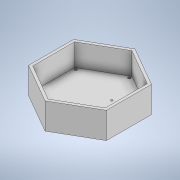
# Autodesk Inventor part: Improved Internal Base
Saved by Autodesk Inventor 2020 (Build 240168000, 168)
## iProperties
Created: 2020-02-13
Part Number: Improved Internal Base
Material: Generic
Document SubType Name: Modeling
Designer: danie
Density: 1 g/cm^3
Appearance: Default
Author: danie
Autodesk Inventor part; units mm, degrees
ref_plane "YZ Plane" through (0, 0, 0) normal (1, 0, 0) x (0, 1, 0)
ref_plane "XZ Plane" through (0, 0, 0) normal (0, 1, 0) x (-1, 0, 0)
ref_plane "XY Plane" through (0, 0, 0) normal (0, 0, 1) x (1, 0, 0)
sketch "Sketch1" plane through (0, 0, 0) normal (0, 1, 0) x (-1, 0, 0)
  line L0 (0, 0) -> (0, -80)
  line L1 (0, -80) -> (69.282, -120)
  line L2 (69.282, -120) -> (138.5641, -80)
  line L3 (138.5641, -80) -> (138.5641, 0)
  line L4 (138.5641, 0) -> (69.282, 40)
  line L5 (69.282, 40) -> (0, 0)
  line L6 (-5, 2.8868) -> (-5, -82.8868)
  line L7 (-5, -82.8868) -> (69.282, -125.7735)
  line L8 (69.282, -125.7735) -> (143.5641, -82.8868)
  line L9 (143.5641, -82.8868) -> (143.5641, 2.8868)
  line L10 (143.5641, 2.8868) -> (69.282, 45.7735)
  line L11 (69.282, 45.7735) -> (-5, 2.8868)
  line L12 (0, 0) -> (-5, 0) construction
  line L13 (-5, 2.8868) -> (0, 0) construction
  dimension "wall" = 80
  dimension "d1" = 80
  dimension "d2" = 80
  dimension "d3" = 80
  dimension "d4" = 80
  dimension "d5" = 80
  dimension "d6" = 120
  dimension "d7" = 120
  dimension "d9" = 120
  dimension "d10" = 120
  dimension "d11" = 120
  dimension "wallThickness" = 5
  dimension "d15" = 5
  dimension "d16" = 148.5641
  constraints: 28 end point, 5 equal length, 2 vertical, 1 parallel, 1 perpendicular, 1 point on line
  measures "wall" distance of L0.start L0.end
  measures "d1" distance of L0.end L1.end
  measures "d2" distance of L1.end L2.end
  measures "d3" distance of L2.end L3.end
  measures "d4" distance of L3.end L4.end
  measures "d5" distance of L0.start L4.end
  measures "d6" angle of L0 L1
  measures "d7" angle of L1 L2
  measures "d9" angle of L2 L3
  measures "d10" angle of L6 L7
  measures "d11" angle of L7 L8
  measures "wallThickness" distance between parallel lines of L6 L0
  measures "d15" distance between parallel lines of L11 L5
  measures "d16" horizontal distance of L6.start L8.end
extrude "Extrusion1" add sketch "Sketch1" along normal blind 7.5 contours L5 L4 L3 L2 L1 L0
extrude "Extrusion2" add sketch "Sketch1" along normal blind 50
sketch "Sketch2" plane through (0, 7.5, 0) normal (0, 1, 0) x (1, 0, 0)
  circle A0 centre (-4.45, 60.955) radius 1.905
  circle A1 centre (-4.45, 19.045) radius 1.905
  line L0 (-4.45, 60.955) -> (-4.45, 19.045) construction
  line L1 (0, 80) -> (0, 0) construction
  line L2 (-4.45, 19.045) -> (-48.935, 19.045) construction
  circle A2 centre (-48.935, 19.045) radius 1.905
  circle A3 centre (-48.935, 60.955) radius 1.905
  line L3 (0, 80) -> (-69.282, 120) projected
  line L4 (0, 80) -> (-1, 80) construction
  dimension "holderRadius" = 3.81
  dimension "d22" = 3.81
  dimension "d23" = 41.91
  dimension "d24" = 4.45
  dimension "d25" = 44.485
  dimension "d26" = 3.81
  dimension "d27" = 3.81
  dimension "d28" = 41.91
  dimension "d29" = 44.485
  dimension "d30" = 1
  dimension "d31" = 19.045
  constraints: 6 end point, 4 centre point, 2 coincident, 1 horizontal, 1 perpendicular, 1 vertical
  measures "holderRadius" diameter of A0
  measures "d22" diameter of A1
  measures "d23" distance of L0.start L0.end
  measures "d24" distance from line of L1 L0.start
  measures "d25" distance of L0.end L2.end
  measures "d26" diameter of A2
  measures "d27" diameter of A3
  measures "d28" distance of L2.end A3.centre
  measures "d29" distance of L0.start A3.centre
  measures "d30" distance of L1.start L4.end
  measures "d31" distance from line of L0.start L4
extrude "Extrusion3" cut sketch "Sketch2" against normal blind 5
sketch "Sketch3" plane through (0, 7.5, 0) normal (0, 1, 0) x (1, 0, 0)
  circle A0 centre (-4.3301, 2.5) radius 2.5
  line L0 (0, 0) -> (0, 80) projected
  line L1 (0, 0) -> (-4.3301, 2.5) construction
  line L2 (0, 0) -> (5, 0) construction
  line L3 (-69.282, -40) -> (-138.5641, 0) construction
  line L4 (-69.282, -40) -> (-69.282, -35) construction
  line L5 (-69.282, -40) -> (-64.282, -40) construction
  line L6 (-138.5641, 80) -> (-138.5641, 0) construction
  line L7 (-138.5641, 0) -> (-134.2339, 2.5) construction
  line L8 (-138.5641, 0) -> (-133.5641, 0) construction
  line L9 (-69.282, 120) -> (-69.282, 115) construction
  line L10 (0, 80) -> (-4.3301, 77.5) construction
  circle A1 centre (-4.3301, 77.5) radius 2.5
  line L11 (-138.5641, 80) -> (-69.282, 120) construction
  circle A2 centre (-134.2339, 2.5) radius 2.5
  line L12 (-138.5641, 80) -> (-134.2339, 77.5) construction
  circle A3 centre (-134.2339, 77.5) radius 2.5
  circle A4 centre (-69.282, 115) radius 2.5
  circle A5 centre (-69.282, -35) radius 2.5
  circle A6 centre (-69.282, -35) radius 1.25
  circle A7 centre (-134.2339, 2.5) radius 1.25
  circle A8 centre (-134.2339, 77.5) radius 1.25
  circle A9 centre (-69.282, 115) radius 1.25
  circle A10 centre (-4.3301, 77.5) radius 1.25
  circle A11 centre (-4.3301, 2.5) radius 1.25
  dimension "holeRad" = 5
  dimension "d35" = 5
  dimension "d36" = 150
  dimension "d37" = 5
  dimension "d38" = 90
  dimension "d39" = 5
  dimension "d40" = 30
  dimension "d42" = 5
  dimension "d43" = 5
  dimension "d44" = 5
  dimension "d45" = 60
  dimension "d47" = 5
  dimension "d48" = 5
  dimension "d49" = 60
  dimension "d50" = 5
  dimension "d51" = 5
  dimension "d52" = 5
  dimension "d53" = 2.5
  dimension "d54" = 2.5
  dimension "d55" = 2.5
  dimension "d56" = 2.5
  dimension "d57" = 2.5
  dimension "d58" = 2.5
  constraints: 18 end point, 15 coincident, 12 centre point, 3 equal length, 3 horizontal, 2 vertical
  measures "holeRad" diameter of A0
  measures "d35" distance of L1.start L1.end
  measures "d36" angle of L2 L1
  measures "d37" distance of L3.start L4.end
  measures "d38" angle of L5 L4
  measures "d39" distance of L3.end L7.end
  measures "d40" angle of L8 L7
  measures "d42" distance of L9.start L9.end
  measures "d43" distance of L0.end L10.end
  measures "d44" diameter of A1
  measures "d45" angle of L0 L10
  measures "d47" diameter of A2
  measures "d48" distance of L6.start L12.end
  measures "d49" angle of L11 L12
  measures "d50" diameter of A3
  measures "d51" diameter of A4
  measures "d52" diameter of A5
  measures "d53" diameter of A6
  measures "d54" diameter of A7
  measures "d55" diameter of A8
  measures "d56" diameter of A9
  measures "d57" diameter of A10
  measures "d58" diameter of A11
extrude "Extrusion4" cut sketch "Sketch3" against normal blind 3.75
extrude "Extrusion5" cut sketch "Sketch3" against normal blind 7.5 contours A6 | A7 | A8 | A9 | A10 | A11
equation "\"d1\" = wall"
equation "\"d2\" = wall"
equation "\"d3\" = wall"
equation "\"d4\" = wall"
equation "\"d5\" = wall"
body "Solid1"
